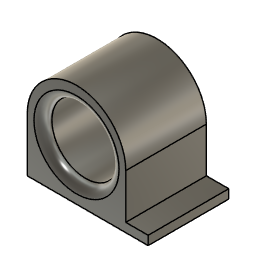
Banner Stand Hook Part B v1 (Autodesk Fusion 360 design; units mm, degrees)
Autodesk Fusion 360 part; units mm, degrees
sketch "Sketch1" plane through (0, 0, 0) normal (0, 0, 1) x (1, 0, 0)
  line L0 (0, 0) -> (27, 0)
  line L1 (27, 0) -> (27, -13)
  line L2 (27, -13) -> (0, -13)
  line L3 (0, -13) -> (0, 0)
  dimension "d1" = 27
  dimension "d2" = 13
  constraint horizontal L0
  constraint vertical L1
  constraint horizontal L2
  constraint vertical L3
  constraint coincident L0.start L3.end
  measures "d1" distance of L0.start L0.end
  measures "d2" distance of L0.start L2.end
extrude "Extrude1" add sketch "Sketch1" along normal blind 0.5
extrude "Extrude2" add 1 faces at (9, -8.6667, 0.5) along direction (0, 0, 1) blind 1.5
sketch "Sketch2" plane through (0, 0, 2) normal (0, 0, 1) x (-1, 0, 0)
  line L0 (0, 13) -> (-27, 13)
  line L1 (-27, 13) -> (-27, 0)
  line L2 (-27, 0) -> (0, 0)
  line L3 (0, 0) -> (0, 13)
  line L4 (0, 13) -> (-22, 13)
  line L5 (-22, 13) -> (-22, -5)
  line L6 (-22, -5) -> (0, -5)
  line L7 (0, -5) -> (0, 13)
  dimension "d7" = 22
  dimension "d8" = 18
  constraint horizontal L4
  constraint vertical L5
  constraint horizontal L6
  constraint vertical L7
  constraint coincident L0.start L3.end
  measures "d7" distance of L0.start L4.end
  measures "d8" distance of L0.start L6.end
extrude "Extrude3" add sketch "Sketch2" along normal blind 21 contours L0 L2 L3 L4 L5 L7 | L2 L5 L6 L7
extrude "Extrude4" add 1 faces at (16.3333, 0, 0.6667) along direction (0, 1, 0) blind 5
sketch "Sketch3" plane through (0, -13, 0) normal (0, -1, 0) x (1, 0, 0)
  line L0 (0, 0) -> (27, 0)
  line L1 (27, 0) -> (27, 2)
  line L2 (27, 2) -> (22, 2)
  line L3 (22, 2) -> (22, 23)
  line L4 (22, 23) -> (0, 23)
  line L5 (0, 23) -> (0, 0)
  circle A0 centre (11, 11.5) radius 7.5
  line L6 (0, 2) -> (22, 2) construction
  line L7 (27.4979, -2) -> (0.4979, -2) construction
  line L8 (-1.5021, 4) -> (29.4979, 4) construction
  dimension "d13" = 15
  dimension "d14" = 6
  dimension "d15" = 7.5
  dimension "d16" = 11
  constraint coincident L5 L6.start
  constraint coincident L2.end L3.start
  constraint perpendicular L5 L7
  constraint horizontal L8
  measures "d13" diameter of A0
  measures "d14" distance of L7 L8
  measures "d15" distance of A0.centre L8
  measures "d16" distance of L3 A0.centre
extrude "Extrude5" cut sketch "Sketch3" against normal blind 15 contours A0
fillet "Fillet1" radius 11 2 edges at (22, -4, 23) (0, -4, 23)
fillet "Fillet2" radius 2 1 edges at (4.0075, -13, 14.2121)
